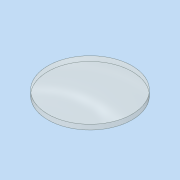
# Autodesk Inventor part: Lense
Saved by Autodesk Inventor 2017 (Build 210142000, 142)
## iProperties
Created: 2018-02-22
Part Number: Lense
Material: Glass
Document SubType Name: Modeling
Designer: Derek Wider
Density: 2.18 g/cm^3
Appearance: Clear
Author: Derek Wider
Autodesk Inventor part; units mm, degrees
ref_plane "YZ Plane" through (0, 0, 0) normal (1, 0, 0) x (0, 1, 0)
ref_plane "XZ Plane" through (0, 0, 0) normal (0, 1, 0) x (-1, 0, 0)
ref_plane "XY Plane" through (0, 0, 0) normal (0, 0, 1) x (1, 0, 0)
sketch "Sketch2" plane through (0, 0, 0) normal (0, 0, 1) x (1, 0, 0)
  line L0 (0, 1) -> (0, 0)
  line L1 (0, 0) -> (4.25, 0)
  line L2 (4.25, 0) -> (4.25, 0.5)
  arc A0 (4.25, 0.5) -> (0, 1) centre (0, -17.3125) ccw
  dimension "d0" = 4.25
  dimension "d1" = 1
  dimension "d2" = 0.5
  constraints: 6 end point, 2 perpendicular, 2 point on circle, 1 centre point, 1 line through centre, 1 vertical
  measures "d0" distance of L0.end L1.end
  measures "d1" distance of L0.start L0.end
  measures "d2" distance of L1.end L2.end
revolve "Revolution1" add sketch "Sketch2" angle 360 about axis through (0, 1, 0) along (0, -1, 0)
body "Solid1"
